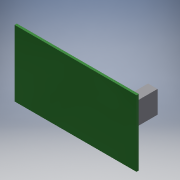
# Autodesk Inventor part: PCB
Saved by Autodesk Inventor 2018 (Build 220112000, 112)
## iProperties
Created: 2018-05-21
Part Number: PCB
Material: Generic
Document SubType Name: Modeling
Designer: David
Density: 1 g/cm^3
Appearance: Default
Author: David
Autodesk Inventor part; units mm, degrees
ref_plane "YZ Plane" through (0, 0, 0) normal (1, 0, 0) x (0, 1, 0)
ref_plane "XZ Plane" through (0, 0, 0) normal (0, 1, 0) x (-1, 0, 0)
ref_plane "XY Plane" through (0, 0, 0) normal (0, 0, 1) x (1, 0, 0)
sketch "Sketch1" plane through (0, 0, 0) normal (0, 1, 0) x (-1, 0, 0)
  line L0 (-80, -43.475) -> (80, -43.475)
  line L1 (80, -43.475) -> (80, 43.475)
  line L2 (80, 43.475) -> (-80, 43.475)
  line L3 (-80, 43.475) -> (-80, -43.475)
  line L4 (-80, -43.475) -> (80, 43.475) construction
  line L5 (80, -43.475) -> (-80, 43.475) construction
  point P0 (0, 0)
  dimension "d0" = 160
  dimension "d1" = 86.95
  constraints: 12 end point, 2 midpoint, 2 parallel, 1 horizontal, 1 perpendicular
  measures "d0" distance of L2.end L1.end
  measures "d1" distance of L1.end L0.end
extrude "Extrusion1" add sketch "Sketch1" along normal blind 3
sketch "Sketch2" plane through (0, 3, 0) normal (0, 1, 0) x (1, 0, 0)
  line L0 (-6.6, 31.775) -> (41.4, 31.775)
  line L1 (41.4, 31.775) -> (41.4, 11.375)
  line L2 (41.4, 11.375) -> (-6.6, 11.375)
  line L3 (-6.6, 11.375) -> (-6.6, 31.775)
  line L4 (80, -43.475) -> (80, 43.475) projected
  line L5 (-80, -43.475) -> (80, -43.475) projected
  line L6 (-75.9, -32.075) -> (-60.6, -32.075)
  line L7 (-60.6, -32.075) -> (-60.6, -9.975)
  line L8 (-60.6, -9.975) -> (-75.9, -9.975)
  line L9 (-75.9, -9.975) -> (-75.9, -32.075)
  line L10 (-80, 43.475) -> (-80, -43.475) projected
  line L11 (-54.5, -32.075) -> (-39.2, -32.075)
  line L12 (-39.2, -32.075) -> (-39.2, -9.975)
  line L13 (-39.2, -9.975) -> (-54.5, -9.975)
  line L14 (-54.5, -9.975) -> (-54.5, -32.075)
  line L15 (-33.1, -32.075) -> (-17.8, -32.075)
  line L16 (-17.8, -32.075) -> (-17.8, -9.975)
  line L17 (-17.8, -9.975) -> (-33.1, -9.975)
  line L18 (-33.1, -9.975) -> (-33.1, -32.075)
  line L19 (57.2, 2.825) -> (69.6, 2.825)
  line L20 (69.6, 2.825) -> (69.6, -26.475)
  line L21 (69.6, -26.475) -> (57.2, -26.475)
  line L22 (57.2, -26.475) -> (57.2, 2.825)
  line L23 (-11.7, -9.975) -> (-11.7, -32.075)
  line L24 (3.6, -9.975) -> (-11.7, -9.975)
  line L25 (3.6, -32.075) -> (3.6, -9.975)
  line L26 (-11.7, -32.075) -> (3.6, -32.075)
  line L27 (31.1, -9.975) -> (31.1, -32.075)
  line L28 (46.4, -9.975) -> (31.1, -9.975)
  line L29 (46.4, -32.075) -> (46.4, -9.975)
  line L30 (31.1, -32.075) -> (46.4, -32.075)
  line L31 (25, -9.975) -> (9.7, -9.975)
  line L32 (9.7, -32.075) -> (25, -32.075)
  line L33 (25, -32.075) -> (25, -9.975)
  line L34 (9.7, -9.975) -> (9.7, -32.075)
  line L35 (80, 43.475) -> (-80, 43.475) projected
  point P0 (0, 0)
  dimension "d6" = 48
  dimension "d7" = 20.4
  dimension "d26" = 15.3
  dimension "d27" = 22.1
  dimension "d29" = 4.1
  dimension "d30" = 15.3
  dimension "d32" = 15.3
  dimension "d36" = 12.4
  dimension "d37" = 29.3
  dimension "d38" = 15.3
  dimension "d42" = 15.3
  dimension "d44" = 15.3
  dimension "d46" = 6.1
  dimension "d47" = 6.1
  dimension "d48" = 6.1
  dimension "d49" = 6.1
  dimension "d50" = 6.1
  dimension "d51" = 11.4
  dimension "d52" = 10.4
  dimension "d53" = 17
  dimension "d54" = 73.4
  dimension "d55" = 11.7
  constraints: 64 end point, 16 parallel, 10 collinear, 8 horizontal, 8 perpendicular
  measures "d6" distance of L1.end L2.end
  measures "d7" distance of L0.end L1.end
  measures "d26" distance of L7.end L8.end
  measures "d27" distance of L6.end L7.end
  measures "d29" distance between parallel lines of L10 L9
  measures "d30" distance of L13.start L14.start
  measures "d32" distance of L17.start L18.start
  measures "d36" distance of L20.end L21.end
  measures "d37" distance of L19.end L20.end
  measures "d38" distance of L24.start L24.end
  measures "d42" distance of L28.start L28.end
  measures "d44" distance of L33.end L34.start
  measures "d46" distance between parallel lines of L7 L14
  measures "d47" distance between parallel lines of L18 L12
  measures "d48" distance between parallel lines of L23 L16
  measures "d49" distance between parallel lines of L25 L34
  measures "d50" distance between parallel lines of L27 L33
  measures "d51" distance between parallel lines of L5 L6
  measures "d52" distance between parallel lines of L4 L20
  measures "d53" distance between parallel lines of L5 L21
  measures "d54" distance between parallel lines of L10 L3
  measures "d55" distance between parallel lines of L35 L0
extrude "Extrusion4" add sketch "Sketch2" along normal blind 10 contours L0 L1 L2 L3 | L9 L8 L7 L6 | L14 L13 L12 L11 | L18 L17 L16 L15 | L19 L20 L21 L22 | L24 L25 L26 L23 | L28 L29 L30 L27 | L33 L32 L34 L31
sketch "Sketch4" plane through (0, 13, 0) normal (0, 1, 0) x (1, 0, 0)
  line L0 (44.5244, 25.526) -> (38.2756, 25.526)
  line L1 (38.2756, 25.526) -> (38.2756, 17.624)
  line L2 (38.2756, 17.624) -> (44.5244, 17.624)
  line L3 (44.5244, 17.624) -> (44.5244, 25.526)
  line L4 (41.4, 11.375) -> (41.4, 31.775) projected
  line L5 (44.5244, 25.526) -> (38.2756, 17.624) construction
  line L6 (38.2756, 25.526) -> (44.5244, 17.624) construction
  point P0 (0, 0)
  point P1 (41.4, 21.575)
  constraints: 12 end point, 3 midpoint, 2 parallel, 1 horizontal, 1 perpendicular
extrude "Extrusion5" add sketch "Sketch4" along normal blind 3
sketch "Sketch5" plane through (0, 3, 0) normal (0, 1, 0) x (1, 0, 0)
  line L0 (65.8, 16.025) -> (50.6, 16.025)
  line L1 (50.6, 16.025) -> (50.6, 10.425)
  line L2 (50.6, 10.425) -> (65.8, 10.425)
  line L3 (65.8, 10.425) -> (65.8, 16.025)
  line L4 (80, 43.475) -> (-80, 43.475) projected
  line L5 (80, -43.475) -> (80, 43.475) projected
  line L6 (65.8, 39.375) -> (50.6, 39.375)
  line L7 (50.6, 39.375) -> (50.6, 33.775)
  line L8 (50.6, 33.775) -> (65.8, 33.775)
  line L9 (65.8, 33.775) -> (65.8, 39.375)
  point P0 (0, 0)
  dimension "d60" = 15.2
  dimension "d61" = 5.6
  dimension "d62" = 27.45
  dimension "d63" = 14.2
  dimension "d64" = 15.2
  dimension "d65" = 5.6
  dimension "d66" = 4.1
  constraints: 16 end point, 4 parallel, 2 horizontal, 2 perpendicular, 1 collinear
  measures "d60" distance of L2.end L1.end
  measures "d61" distance of L0.end L1.end
  measures "d62" distance between parallel lines of L4 L0
  measures "d63" distance between parallel lines of L5 L3
  measures "d64" distance of L8.end L7.end
  measures "d65" distance of L6.end L7.end
  measures "d66" distance between parallel lines of L4 L6
extrude "Extrusion6" add sketch "Sketch5" along normal blind 8.5
sketch "Sketch6" plane through (0, 13, 0) normal (0, 1, 0) x (1, 0, 0)
  line L0 (57.2, -26.475) -> (69.6, -26.475) projected
  line L1 (69.6, -26.475) -> (57.2, -26.475)
  line L2 (57.2, -26.475) -> (57.2, 2.825)
  line L3 (57.2, 2.825) -> (69.6, 2.825)
  line L4 (69.6, 2.825) -> (69.6, -26.475)
  point P0 (0, 0)
  constraints: 8 end point, 2 parallel, 1 horizontal, 1 perpendicular
extrude "Extrusion7" add sketch "Sketch6" along normal blind 25
body "Solid1"
